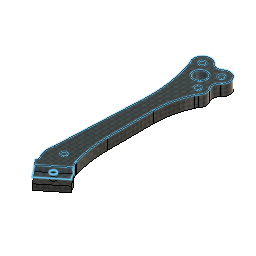
T_v7_Shorty_Arm_5_Inch_6mm (Autodesk Fusion 360 design; units mm, degrees)
Autodesk Fusion 360 part; units mm, degrees
sketch "T_v1_Arm_5_Inch_Shorty_6mm_or_5mm_4x" plane through (0, 0, 0) normal (0, 0, 1) x (1, 0, 0)
  arc A0 (-225.6533, 220.9552) -> (-220.6279, 220.4722) centre (-222.8873, 223.3495) ccw
  arc A1 (-230.3335, 140.9887) -> (-229.5344, 133.9506) centre (-220.257, 138.5683) ccw
  arc A2 (-217.3945, 140.1231) -> (-217.1516, 139.4711) centre (-212.5989, 141.5382) ccw
  line L0 (-215.5389, 136.8403) -> (-226.8186, 127.742)
  arc A3 (-215.5389, 136.8403) -> (-214.3199, 135.521) centre (-209.8871, 140.8396) ccw
  arc A4 (-215.7785, 202.7474) -> (-216.6488, 201.3936) centre (-212.0626, 199.402) ccw
  arc A5 (-215.0172, 213.5689) -> (-220.6279, 220.4722) centre (-217.8805, 216.9734) ccw
  arc A6 (-220.2406, 159.5651) -> (-217.3945, 140.1231) centre (-150.6263, 159.8267) ccw
  arc A7 (-215.7785, 202.7474) -> (-215.5657, 208.4451) centre (-219.0846, 205.7238) ccw
  circle A8 centre (-217.8805, 216.9734) radius 1.5
  arc A9 (-228.9289, 130.3582) -> (-229.2844, 133.4743) centre (-231.6499, 131.6261) ccw
  circle A10 centre (-224.0861, 140.4692) radius 1.45
  circle A11 centre (-218.5249, 129.3701) radius 1.45
  arc A12 (-216.6488, 201.3936) -> (-220.3306, 183.5032) centre (-175.8354, 183.6704) ccw
  arc A13 (-225.6533, 220.9552) -> (-232.9473, 215.8914) centre (-229.1297, 218.1776) ccw
  arc A14 (-229.5344, 133.9506) -> (-229.2844, 133.4743) centre (-228.5434, 134.167) ccw
  circle A15 centre (-219.0847, 205.7238) radius 1.5
  arc A16 (-211.6169, 132.1699) -> (-210.5855, 130.6992) centre (-205.2604, 135.5308) ccw
  arc A17 (-217.1516, 139.4711) -> (-215.5389, 136.8403) centre (-205.7671, 144.6403) ccw
  line L1 (-221.8653, 121.601) -> (-228.9289, 130.3582)
  circle A18 centre (-224.0878, 211.9497) radius 3.5
  circle A19 centre (-218.5249, 129.3701) radius 1.45
  arc A20 (-228.2024, 185.7996) -> (-232.5238, 214.992) centre (-304.8727, 189.366) ccw
  line L2 (-220.2406, 159.5651) -> (-220.3306, 183.5032)
  circle A21 centre (-229.1297, 218.1776) radius 1.5
  arc A22 (-232.5238, 214.992) -> (-232.9473, 215.8914) centre (-237.2369, 213.3226) ccw
  arc A23 (-211.6169, 132.1699) -> (-214.3199, 135.521) centre (-218.6052, 129.2988) ccw
  line L3 (-210.5855, 130.6992) -> (-221.8653, 121.601)
  arc A24 (-215.0172, 213.5689) -> (-215.5657, 208.4451) centre (-212.6223, 210.7213) ccw
  arc A25 (-228.2024, 185.7996) -> (-230.2645, 141.4764) centre (17543.3039, -663.1993) ccw
  arc A26 (-230.3335, 140.9887) -> (-230.2645, 141.4764) centre (-232.8519, 141.5936) ccw
extrude "Extrude1" add sketch "T_v1_Arm_5_Inch_Shorty_6mm_or_5mm_4x" against normal blind 5.5 makes body 1
extrude "Extrude2" cut sketch "T_v1_Arm_5_Inch_Shorty_6mm_or_5mm_4x" against normal blind 2.75 contours L0 A3 A16 L1 A23 L3 bodies 1
extrude "Extrude3" add sketch "T_v1_Arm_5_Inch_Shorty_6mm_or_5mm_4x" against normal blind 6 separate body makes body 2
extrude "Extrude4" cut sketch "T_v1_Arm_5_Inch_Shorty_6mm_or_5mm_4x" against normal blind 3 contours L0 A3 A16 L1 A23 L3 bodies 2
hidden bodies 1
named bodies: "5 Inch Shorty 5.5mm 7.92gr", "5  Shorty Arm 6mm"
